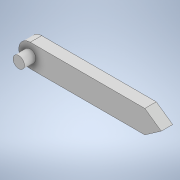
# Autodesk Inventor part: Punta de flecha
Saved by Autodesk Inventor 2020 (Build 240168000, 168)
## iProperties
Created: 2020-11-30
Part Number: Punta de flecha
Material: Generic
Document SubType Name: Modeling
Designer: Daniel
Density: 1 g/cm^3
Appearance: Default
Author: Daniel
Autodesk Inventor part; units mm, degrees
ref_plane "YZ Plane" through (0, 0, 0) normal (1, 0, 0) x (0, 1, 0)
ref_plane "XZ Plane" through (0, 0, 0) normal (0, 1, 0) x (-1, 0, 0)
ref_plane "XY Plane" through (0, 0, 0) normal (0, 0, 1) x (1, 0, 0)
sketch "Sketch1" plane through (0, 0, 0) normal (0, 0, 1) x (1, 0, 0)
  line L0 (0, 0) -> (254, 0)
  line L1 (0, 50.8) -> (254, 50.8)
  arc A0 (0, 50.8) -> (0, 0) centre (0, 25.4) ccw
  line L2 (254, 50.8) -> (290.3943, 25.4)
  line L3 (290.3943, 25.4) -> (254, 0)
  circle A1 centre (0, 25.4) radius 12.7
  dimension "d0" = 254
  dimension "d1" = 254
  dimension "d2" = 50.8
  dimension "d3" = 25.4
  dimension "d4" = 25.4
  constraints: 8 end point, 2 centre point, 2 horizontal, 2 point on circle, 2 tangent, 1 coincident
  measures "d0" distance of L0.start L0.end
  measures "d1" distance of L1.start L1.end
  measures "d2" distance between parallel lines of L0 L1
  measures "d3" distance from line of L0 L2.end
  measures "d4" diameter of A1
extrude "Extrusion1" add sketch "Sketch1" along normal blind 25.4 contours A0 L1 L2 L3 L0 | A1
sketch "Sketch2" plane through (0, 0, 25.4) normal (0, 0, 1) x (1, 0, 0)
  circle A0 centre (0, 25.4) radius 12.7
  arc A1 (0, 50.8) -> (0, 0) centre (0, 25.4) ccw projected
  dimension "d7" = 25.4
  constraints: 1 centre point, 1 concentric
  measures "d7" diameter of A0
extrude "Extrusion2" add sketch "Sketch2" along normal blind 25.4
body "Solid1"
